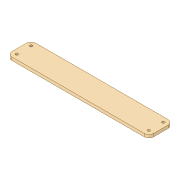
# Autodesk Inventor part: supportPlate
Saved by Autodesk Inventor 2017 (Build 210142000, 142)
## iProperties
Created: 2017-03-01
Part Number: supportPlate
Material: ABS Plastic
Document SubType Name: Modeling
Designer: sawaiz
Density: 1.06 g/cm^3
Appearance: Smooth - Off-White
Author: sawaiz
Autodesk Inventor part; units mm, degrees
ref_plane "YZ Plane" through (0, 0, 0) normal (1, 0, 0) x (0, 1, 0)
ref_plane "XZ Plane" through (0, 0, 0) normal (0, 1, 0) x (-1, 0, 0)
ref_plane "XY Plane" through (0, 0, 0) normal (0, 0, 1) x (1, 0, 0)
sketch "Sketch1" plane through (0, 0, 0) normal (0, 1, 0) x (-1, 0, 0)
  line L0 (148, 25) -> (-148, 25)
  line L1 (-148, 25) -> (-148, -25)
  line L2 (-148, -25) -> (148, -25)
  line L3 (148, -25) -> (148, 25)
  line L4 (148, 25) -> (-148, -25) construction
  line L5 (-148, 25) -> (148, -25) construction
  point P0 (0, 0)
  dimension "d0" = 296
  dimension "d1" = 50
  constraints: 12 end point, 2 midpoint, 2 parallel, 1 horizontal, 1 perpendicular
  measures "d0" distance of L2.end L1.end
  measures "d1" distance of L1.end L0.end
extrude "Extrusion1" add sketch "Sketch1" along normal mid plane 6.35
fillet "Fillet1" radius 10 4 edges at (-148, 0, 25) (-148, 0, -25) (148, 0, -25) (148, 0, 25)
sketch "Sketch2" plane through (0, 3.175, 0) normal (0, 1, 0) x (1, 0, 0)
  arc A0 (138, -25) -> (148, -15) centre (138, -15) ccw projected
  line L0 (138, 25) -> (-138, 25) projected
  arc A1 (-138, 25) -> (-148, 15) centre (-138, 15) ccw projected
  line L1 (-138, -25) -> (138, -25) projected
  line L2 (148, -15) -> (148, 15) projected
  arc A2 (148, 15) -> (138, 25) centre (138, 15) ccw projected
  line L3 (-148, 15) -> (-148, -15) projected
  arc A3 (-148, -15) -> (-138, -25) centre (-138, -15) ccw projected
  point P0 (0, 0)
  dimension "d6" = 10
  dimension "d14" = 10
  measures "d6" distance from line of L1 point (-138, -15)
  measures "d14" distance from line of L3 point (-138, -15)
hole "Hole1" at (-138, 3.175, 15) direction (0, -1, 0) diameter 5.5118 end through all clearance for "Socket Head Cap Screw" size "M5" standard "Ansi Metric M Profile"
mirror "Mirror1" about plane through (0, 0, 0) normal (0, 0, 1) of "Hole1"
mirror "Mirror2" about plane through (0, 0, 0) normal (1, 0, 0) of "Hole1", "Mirror1"
equation "\"d1\" = supportPlateWidth"
equation "\"d2\" = supportPlateThickness"
equation "\"d4\" = supportPlateFillet"
equation "\"supportPlateThickness\" = 6.35"
equation "\"supportPlateWidth\" = 50"
equation "\"plateFillet\" = 12.7"
equation "\"supportplateFillet\" = 12.7"
equation "\"separation\" = 35"
equation "\"centerVerticalRatio\" = 0.3"
equation "\"supportPlateFillet\" = 10"
body "Solid1"
